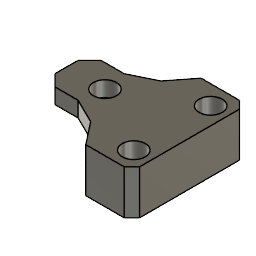
board mount 2x (Autodesk Fusion 360 design; units mm, degrees)
Autodesk Fusion 360 part; units mm, degrees
sketch "Szkic1" plane through (0, 0, 0) normal (0, 0, 1) x (1, 0, 0)
  line L0 (0, -37) -> (0, 37)
  circle A0 centre (7.5, 0) radius 2.1
  line L1 (0, 5) -> (0, -5)
  line L2 (-20, -5) -> (-20, 5)
  circle A1 centre (-10, 0) radius 3
  line L3 (12, 15) -> (12, -15)
  line L4 (12, -15) -> (0, -15)
  line L5 (12, 15) -> (0, 15)
  circle A2 centre (7.5, -10) radius 3
  circle A3 centre (7.5, 10) radius 3
  circle A4 centre (7.5, 10) radius 1.75
  circle A5 centre (7.5, -10) radius 1.75
  line L6 (-20, -5) -> (-20, -6)
  line L7 (-20, -6) -> (0, -6)
  line L8 (0, 6) -> (-20, 6)
  line L9 (-20, 6) -> (-20, 5)
  line L10 (0, 15) -> (-7, 6)
  line L11 (-7, -6) -> (0, -15)
  dimension "d4" = 6
  dimension "d5" = 6
  dimension "d6" = 6
  dimension "d7" = 3.5
  dimension "d8" = 3.5
  constraint coincident L0 L1.end
  constraint parallel L0 L1
  constraint vertical L3
  constraint coincident L0 L4.end
  constraint perpendicular L0 L4
  constraint perpendicular L3 L5
  constraint coincident L0 L7.end
  constraint perpendicular L0 L7
  constraint coincident L0 L8.start
  constraint perpendicular L0 L8
  constraint coincident L8 L10.end
  constraint coincident L7 L11.start
  measures "d4" diameter of A1
  measures "d5" diameter of A2
  measures "d6" diameter of A3
  measures "d7" diameter of A4
  measures "d8" diameter of A5
extrude "Wyciągnięcie proste1" add sketch "Szkic1" along normal blind 4 contours L0 L7 L11 | L0 L1 L2 L6 L7 L8 L9 | L0 L8 L10 makes body 1
extrude "Wyciągnięcie proste2" add sketch "Szkic1" against normal blind 7.5 separate body contours L0 L1 L3 L4 L5 makes body 2
extrude "Wyciągnięcie proste3" add sketch "Szkic1" against normal blind 7.5 contours A2 | A3 bodies 2
extrude "Wyciągnięcie proste4" add sketch "Szkic1" against normal blind 7.5 contours A0 bodies 2
extrude "Wyciągnięcie proste5" cut sketch "Szkic1" against normal blind 3 contours A2 bodies 2
extrude "Wyciągnięcie proste6" cut sketch "Szkic1" against normal blind 3 contours A3 bodies 2
sketch "Szkic2" plane through (0, -15, 0) normal (0, -1, 0) x (1, 0, 0)
  line L0 (12, 0) -> (0, 0)
  line L1 (0, 0) -> (0, -7.5)
  line L2 (0, -7.5) -> (12, -7.5)
  line L3 (12, -7.5) -> (12, 0)
  line L4 (0, 4) -> (0, 0)
  line L5 (0, 0) -> (3, 0)
  line L6 (3, 0) -> (3, 4)
  line L7 (3, 4) -> (0, 4)
  line L8 (3, 4) -> (7, 0)
  point P0 (0, 4)
  constraint perpendicular L4 L5
  constraint parallel L4 L6
  constraint parallel L5 L7
  constraint coincident L0.end L1.start
  constraint perpendicular L0 L4
  constraint coincident P0 L4.start
  constraint coincident L0 L8.end
extrude "Wyciągnięcie proste7" add sketch "Szkic2" against normal blind 30 contours L0 L6 L8 | L0 L4 L5 L6 L7 bodies 1 2
extrude "Wyciągnięcie proste8" cut sketch "Szkic1" along normal blind 5.5 contours A2 | A3 bodies 1 makes body 3 at (6.8281, 9.4547, 0.1719) makes body 4 at (6.8281, -10.5453, 0.1719)
extrude "Wyciągnięcie proste9" cut sketch "Szkic2" against normal blind 52 contours L0 L6 L8 | L0 L4 L5 L6 L7 bodies 1 3 4
extrude "Wyciągnięcie proste10" add 1 faces at (0, 5, 1.3333) along direction (1, 0, 0) blind 12 on bodies 1 bodies 1 3 4
extrude "Wyciągnięcie proste11" cut sketch "Szkic1" along normal blind 8 contours A2 | A3 | A4 | A5 bodies 1
extrude "Wyciągnięcie proste12" add sketch "Szkic1" against normal blind 3 contours A2 | A3 | A4 | A5 bodies 1
extrude "Wyciągnięcie proste13" cut sketch "Szkic1" against normal blind 2.8 contours A2 | A3 | A4 | A5 bodies 1
chamfer "Fazowanie1" distance 2 angle 45 1 edges at (12, -15, -1.75) on bodies 1
chamfer "Fazowanie2" distance 2 angle 45 1 edges at (12, 15, -1.75) on bodies 1
chamfer "Fazowanie3" distance 3 angle 45 1 edges at (-20, -6, 2) on bodies 1
sketch "Szkic3" plane through (0, 0, 4) normal (0, 0, 1) x (-1, 0, 0)
  circle A0 centre (10, 0) radius 3
  line L0 (20, 3) -> (17, 6)
  line L1 (17, 6) -> (7, 6)
  line L2 (7, 6) -> (0, 15)
  line L3 (0, 15) -> (-10, 15)
  line L4 (-10, 15) -> (-12, 13)
  line L5 (-12, 13) -> (-12, -13)
  line L6 (-12, -13) -> (-10, -15)
  line L7 (-10, -15) -> (0, -15)
  line L8 (0, -15) -> (7, -6)
  line L9 (7, -6) -> (20, -6)
  line L10 (20, -6) -> (20, -5)
  line L11 (20, -5) -> (20, 3)
  circle A1 centre (-7.5, -10) radius 3
  circle A2 centre (-7.5, 10) radius 3
  line L12 (20, -3) -> (17, -6)
  constraint coincident L11 L12.start
  constraint coincident L9 L12.end
extrude "Wyciągnięcie proste14" cut sketch "Szkic3" against normal blind 9 contours L9 L10 L11 L12 bodies 1
chamfer "Fazowanie4" distance 4 angle 45 1 edges at (-7, -6, 2) on bodies 1
chamfer "Fazowanie5" distance 4 angle 45 1 edges at (-7, 6, 2) on bodies 1
